Autodesk Inventor part; units mm, degrees
(part 2 of 2)
  point P149 (-1.693, 40.4752)
  point P150 (-1.6779, 40.4117)
  point P151 (-1.6594, 40.3487)
  point P152 (-5.9644, 41.4834)
  point P153 (-3.9838, 41.7202)
  point P154 (-4.0844, 40.3041)
  point P155 (-4.0904, 40.2391)
  point P156 (-4.0997, 40.1742)
  point P157 (-4.7872, 40.0384)
  point P158 (-5.5328, 40.131)
  point P159 (-5.5116, 40.0692)
  point P160 (-5.4872, 40.0083)
  point P161 (-9.8807, 40.7286)
  point P162 (-7.9315, 41.1526)
  point P163 (-7.8971, 39.7334)
  point P164 (-7.8968, 39.6681)
  point P165 (-7.9, 39.6025)
  point P166 (-9.3224, 39.4233)
  point P167 (-9.2955, 39.3638)
  point P168 (-9.2654, 39.3055)
  point P169 (-13.7074, 39.605)
  point P170 (-11.8074, 40.2124)
  point P171 (-11.6382, 38.8028)
  point P172 (-11.6318, 38.7378)
  point P173 (-11.6287, 38.6723)
  point P174 (-12.278, 38.4088)
  point P175 (-13.0276, 38.3587)
  point P176 (-12.9952, 38.302)
  point P177 (-12.9597, 38.2468)
  point P178 (-17.41, 38.1227)
  point P179 (-15.5764, 38.9079)
  point P180 (-15.274, 37.5208)
  point P181 (-15.2614, 37.4567)
  point P182 (-15.252, 37.3918)
  point P183 (-15.8734, 37.0678)
  point P184 (-16.6148, 36.9466)
  point P185 (-16.5772, 36.8933)
  point P186 (-16.5366, 36.8417)
  point P187 (-20.955, 36.2951)
  point P188 (-19.2043, 37.2511)
  point P189 (-18.7714, 35.899)
  point P190 (-18.7528, 35.8364)
  point P191 (-18.7373, 35.7727)
  point P192 (-19.325, 35.3911)
  point P193 (-20.0516, 35.2)
  point P194 (-20.009, 35.1505)
  point P195 (-19.9637, 35.103)
  point P196 (-24.3102, 34.1389)
  point P197 (-22.6583, 35.2569)
  point P198 (-22.0988, 33.9521)
  point P199 (-22.0743, 33.8916)
  dimension "d1" = 14.5
  dimension "d2" = 10.4934
  dimension "d12" = 75.5
  dimension "d15" = 40.3225
  dimension "d16" = 75.5
  dimension "d17" = 40.3225
  dimension "d18" = 75.5
  dimension "d19" = 40.3225
  dimension "d20" = 75.5
  dimension "d21" = 40.3225
  dimension "d23" = 10.4934
  dimension "d24" = 4.2774
  dimension "d26" = 1.364
  dimension "d27" = 14.7708
  dimension "d30" = 360
  constraints: 338 point on circle, 136 centre point, 36 end point, 7 symmetric about line, 6 point on line, 2 coincident, 2 equal length, 1 collinear, 1 horizontal, 1 horizontal alignment, 1 perpendicular, 1 tangent, 1 vertical, 2598 other
  measures "d1" angle of L0 L1
  measures "d2" distance of L1.end L0.end
  measures "d12" angle of L3 L5
  measures "d15" distance from line of point (0, 0) L3
  measures "d17" distance from line of point (0, 0) L6
  measures "d18" angle of L9 L10
  measures "d19" distance from line of point (0, 0) L9
  measures "d20" angle of L12 L13
  measures "d21" distance from line of L0.start L12
  measures "d26" angle of L0 L17
  measures "d27" distance of L16.start L16.end
extrude "Extrusion1" add sketch "Sketch1" along normal blind 9.525 contours S1 S0 A4 A7 S2 S3 A3 S260 S263 A137 A136 S262 S261 S256 S259 A135 A134 S258 S257 S252 S255 A133 A132 S254 S253 S248 S251 A131 A130 S250 S249 S244 S247 A129 A128 S246 S245 S240 S243 A127 A126 S242 S241 S236 S239 A125 A124 S238 S237 S232 S235 A123 A122 S234 S233 S228 S231 A121 A120 S230 S229 S224 S227 A119 A118 S226 S225 S220 S223 A117 A116 S222 S221 S216 S219 A115 A114 S218 S217 S212 S215 A113 A112 S214 S213 S208 S211 A111 A110 S210 S209 S204 S207 A109 A108 S206 S205 S200 S203 A107 A106 S202 S201 S196 S199 A105 A104 S198 S197 S192 S195 A103 A102 S194 S193 S188 S191 A101 A100 S190 S189 S184 S187 A99 A98 S186 S185 S180 S183 A97 A96 S182 S181 S176 S179 A95 A94 S178 S177 S172 S175 A93 A92 S174 S173 S168 S171 A91 A90 S170 S169 S164 S167 A89 A88 S166 S165 S160 S163 A87 A86 S162 S161 S156 S159 A85 A84 S158 S157 S152 S155 A83 A82 S154 S153 S148 S151 A81 A80 S150 S149 S144 S147 A79 A78 S146 S145 S140 S143 A77 A76 S142 S141 S136 S139 A75 A74 S138 S137 S132 S135 A73 A72 S134 S133 S128 S131 A71 A70 S130 S129 S124 S127 A69 A68 S126 S125 S120 S123 A67 A66 S122 S121 S116 S119 A65 A64 S118 S117 S112 S115 A63 A62 S114 S113 S108 S111 A61 A60 S110 S109 S104 S107 A59 A58 S106 S105 S100 S103 A57 A56 S102 S101 S96 S99 A55 A54 S98 S97 S92 S95 A53 A52 S94 S93 S88 S91 A51 A50 S90 S89 S84 S87 A49 A48 S86 S85 S80 S83 A47 A46 S82 S81 S76 S79 A45 A44 S78 S77 S72 S75 A43 A42 S74 S73 S68 S71 A41 A40 S70 S69 S64 S67 A39 A38 S66 S65 S60 S63 A37 A36 S62 S61 S56 S59 A35 A34 S58 S57 S52 S55 A33 A32 S54 S53 S48 S51 A31 A30 S50 S49 S44 S47 A29 A28 S46 S45 S40 S43 A27 A26 S42 S41 S36 S39 A25 A24 S38 S37 S32 S35 A23 A22 S34 S33 S28 S31 A21 A20 S30 S29 S24 S27 A19 A18 S26 S25 S20 S23 A17 A16 S22 S21 S16 S19 A15 A14 S18 S17 S12 S15 A13 A12 S14 S13 S8 S11 A11 A10 S10 S9 S4 S7 A9 A8 S6 S5
sketch "Sketch2" plane through (0, 9.525, 0) normal (0, 1, 0) x (1, 0, 0)
  line L0 (-6.35, 3.6662) -> (0, 7.3323)
  line L1 (0, 7.3323) -> (6.35, 3.6662)
  line L2 (6.35, 3.6662) -> (6.35, -3.6662)
  line L3 (6.35, -3.6662) -> (0, -7.3323)
  line L4 (0, -7.3323) -> (-6.35, -3.6662)
  line L5 (-6.35, -3.6662) -> (-6.35, 3.6662)
  point P0 (0, 0)
  point P1 (0, 0)
  dimension "d34" = 12.7
  constraints: 12 end point, 1 coincident, 1 vertical alignment, 13 other
  measures "d34" distance between parallel lines of L2 L5
sketch "Sketch4" plane through (0, 0, 0) normal (0, -1, 0) x (1, 0, 0)
  arc A0 (-40.3225, -0.2901) -> (-40.2906, -1.6288) centre (0, 0) ccw projected
  arc A1 (-43.11, -2.4585) -> (-43.021, -3.7017) centre (0, 0) ccw projected
  arc A2 (-40.1123, -4.1217) -> (-39.9534, -5.4513) centre (0, 0) ccw projected
  arc A3 (-42.6811, -6.5452) -> (-42.4744, -7.7743) centre (0, 0) ccw projected
  arc A4 (-39.5389, -7.916) -> (-39.2543, -9.2244) centre (0, 0) ccw projected
  arc A5 (-41.8656, -10.5727) -> (-41.543, -11.7766) centre (0, 0) ccw projected
  arc A6 (-38.6074, -11.6385) -> (-38.1997, -12.914) centre (0, 0) ccw projected
  arc A7 (-40.6711, -14.5044) -> (-40.2355, -15.6722) centre (0, 0) ccw projected
  arc A8 (-37.3263, -15.2557) -> (-36.7992, -16.4867) centre (0, 0) ccw projected
  arc A9 (-39.1082, -18.3048) -> (-38.5636, -19.4258) centre (0, 0) ccw projected
  arc A10 (-35.7071, -18.7347) -> (-35.0654, -19.91) centre (0, 0) ccw projected
  arc A11 (-37.1911, -21.9393) -> (-36.5424, -23.0036) centre (0, 0) ccw projected
  arc A12 (-33.7646, -22.0441) -> (-33.014, -23.153) centre (0, 0) ccw projected
  arc A13 (-34.9372, -25.3752) -> (-34.1903, -26.373) centre (0, 0) ccw projected
  arc A14 (-31.5163, -25.1538) -> (-30.6637, -26.1864) centre (0, 0) ccw projected
  arc A15 (-32.367, -28.5813) -> (-31.5286, -29.5036) centre (0, 0) ccw projected
  arc A16 (-28.9825, -28.0357) -> (-28.0357, -28.9825) centre (0, 0) ccw projected
  arc A17 (-29.5036, -31.5286) -> (-28.5813, -32.367) centre (0, 0) ccw projected
  arc A18 (-26.1864, -30.6637) -> (-25.1538, -31.5163) centre (0, 0) ccw projected
  arc A19 (-26.373, -34.1903) -> (-25.3752, -34.9372) centre (0, 0) ccw projected
  arc A20 (-23.153, -33.014) -> (-22.0441, -33.7646) centre (0, 0) ccw projected
  arc A21 (-23.0036, -36.5424) -> (-21.9393, -37.1911) centre (0, 0) ccw projected
  arc A22 (-19.91, -35.0654) -> (-18.7347, -35.7071) centre (0, 0) ccw projected
  arc A23 (-19.4258, -38.5636) -> (-18.3048, -39.1082) centre (0, 0) ccw projected
  arc A24 (-16.4867, -36.7992) -> (-15.2557, -37.3263) centre (0, 0) ccw projected
  arc A25 (-15.6722, -40.2355) -> (-14.5044, -40.6711) centre (0, 0) ccw projected
  arc A26 (-12.914, -38.1997) -> (-11.6385, -38.6074) centre (0, 0) ccw projected
  arc A27 (-11.7766, -41.543) -> (-10.5727, -41.8656) centre (0, 0) ccw projected
  arc A28 (-9.2244, -39.2543) -> (-7.916, -39.5389) centre (0, 0) ccw projected
  arc A29 (-7.7743, -42.4744) -> (-6.5452, -42.6811) centre (0, 0) ccw projected
  arc A30 (-5.4513, -39.9534) -> (-4.1217, -40.1123) centre (0, 0) ccw projected
  arc A31 (-3.7017, -43.021) -> (-2.4585, -43.11) centre (0, 0) ccw projected
  arc A32 (-1.6288, -40.2906) -> (-0.2901, -40.3225) centre (0, 0) ccw projected
  arc A33 (0.4045, -43.1781) -> (1.6505, -43.1484) centre (0, 0) ccw projected
  arc A34 (2.2084, -40.263) -> (3.5441, -40.1675) centre (0, 0) ccw projected
  arc A35 (4.507, -42.9441) -> (5.7445, -42.7962) centre (0, 0) ccw projected
  arc A36 (6.0257, -39.8708) -> (7.3462, -39.6487) centre (0, 0) ccw projected
  arc A37 (8.5687, -42.3213) -> (9.7866, -42.0563) centre (0, 0) ccw projected
  arc A38 (9.7883, -39.1175) -> (11.0818, -38.7709) centre (0, 0) ccw projected
  arc A39 (12.5528, -41.3151) -> (13.7399, -40.9356) centre (0, 0) ccw projected
  arc A40 (13.4624, -38.0099) -> (14.717, -37.5419) centre (0, 0) ccw projected
  arc A41 (16.4232, -39.9348) -> (17.5689, -39.4442) centre (0, 0) ccw projected
  arc A42 (17.0145, -36.5581) -> (18.219, -35.973) centre (0, 0) ccw projected
  arc A43 (20.1449, -38.1929) -> (21.2388, -37.5956) centre (0, 0) ccw projected
  arc A44 (20.4125, -34.7752) -> (21.5559, -34.0783) centre (0, 0) ccw projected
  arc A45 (23.6841, -36.1051) -> (24.7163, -35.4065) centre (0, 0) ccw projected
  arc A46 (23.6257, -32.6774) -> (24.6977, -31.875) centre (0, 0) ccw projected
  arc A47 (27.0089, -33.6903) -> (27.97, -32.8967) centre (0, 0) ccw projected
  arc A48 (26.6249, -30.2837) -> (27.6157, -29.383) centre (0, 0) ccw projected
  arc A49 (30.089, -30.9703) -> (30.9703, -30.089) centre (0, 0) ccw projected
  arc A50 (29.383, -27.6157) -> (30.2837, -26.6249) centre (0, 0) ccw projected
  arc A51 (32.8967, -27.97) -> (33.6903, -27.0089) centre (0, 0) ccw projected
  arc A52 (31.875, -24.6977) -> (32.6774, -23.6257) centre (0, 0) ccw projected
  arc A53 (35.4065, -24.7163) -> (36.1051, -23.6841) centre (0, 0) ccw projected
  arc A54 (34.0783, -21.5559) -> (34.7752, -20.4125) centre (0, 0) ccw projected
  arc A55 (37.5956, -21.2388) -> (38.1929, -20.1449) centre (0, 0) ccw projected
  arc A56 (35.973, -18.219) -> (36.5581, -17.0145) centre (0, 0) ccw projected
  arc A57 (39.4442, -17.5689) -> (39.9348, -16.4232) centre (0, 0) ccw projected
  arc A58 (37.5419, -14.717) -> (38.0099, -13.4624) centre (0, 0) ccw projected
  arc A59 (40.9356, -13.7399) -> (41.3151, -12.5528) centre (0, 0) ccw projected
  arc A60 (38.7709, -11.0818) -> (39.1175, -9.7883) centre (0, 0) ccw projected
  arc A61 (42.0563, -9.7866) -> (42.3213, -8.5687) centre (0, 0) ccw projected
  arc A62 (39.6487, -7.3462) -> (39.8708, -6.0257) centre (0, 0) ccw projected
  arc A63 (42.7962, -5.7445) -> (42.9441, -4.507) centre (0, 0) ccw projected
  arc A64 (40.1675, -3.5441) -> (40.263, -2.2084) centre (0, 0) ccw projected
  arc A65 (43.1484, -1.6505) -> (43.1781, -0.4045) centre (0, 0) ccw projected
  arc A66 (40.3225, 0.2901) -> (40.2906, 1.6288) centre (0, 0) ccw projected
  arc A67 (43.11, 2.4585) -> (43.021, 3.7017) centre (0, 0) ccw projected
  arc A68 (40.1123, 4.1217) -> (39.9534, 5.4513) centre (0, 0) ccw projected
  arc A69 (42.6811, 6.5452) -> (42.4744, 7.7743) centre (0, 0) ccw projected
  arc A70 (39.5389, 7.916) -> (39.2543, 9.2244) centre (0, 0) ccw projected
  arc A71 (41.8656, 10.5727) -> (41.543, 11.7766) centre (0, 0) ccw projected
  arc A72 (38.6074, 11.6385) -> (38.1997, 12.914) centre (0, 0) ccw projected
  arc A73 (40.6711, 14.5044) -> (40.2355, 15.6722) centre (0, 0) ccw projected
  arc A74 (37.3263, 15.2557) -> (36.7992, 16.4867) centre (0, 0) ccw projected
  arc A75 (39.1082, 18.3048) -> (38.5636, 19.4258) centre (0, 0) ccw projected
  arc A76 (35.7071, 18.7347) -> (35.0654, 19.91) centre (0, 0) ccw projected
  arc A77 (37.1911, 21.9393) -> (36.5424, 23.0036) centre (0, 0) ccw projected
  arc A78 (33.7646, 22.0441) -> (33.014, 23.153) centre (0, 0) ccw projected
  arc A79 (34.9372, 25.3752) -> (34.1903, 26.373) centre (0, 0) ccw projected
  arc A80 (31.5163, 25.1538) -> (30.6637, 26.1864) centre (0, 0) ccw projected
  arc A81 (32.367, 28.5813) -> (31.5286, 29.5036) centre (0, 0) ccw projected
  arc A82 (28.9825, 28.0357) -> (28.0357, 28.9825) centre (0, 0) ccw projected
  arc A83 (29.5036, 31.5286) -> (28.5813, 32.367) centre (0, 0) ccw projected
  arc A84 (26.1864, 30.6637) -> (25.1538, 31.5163) centre (0, 0) ccw projected
  arc A85 (26.373, 34.1903) -> (25.3752, 34.9372) centre (0, 0) ccw projected
  arc A86 (23.153, 33.014) -> (22.0441, 33.7646) centre (0, 0) ccw projected
  arc A87 (23.0036, 36.5424) -> (21.9393, 37.1911) centre (0, 0) ccw projected
  arc A88 (19.91, 35.0654) -> (18.7347, 35.7071) centre (0, 0) ccw projected
  arc A89 (19.4258, 38.5636) -> (18.3048, 39.1082) centre (0, 0) ccw projected
  arc A90 (16.4867, 36.7992) -> (15.2557, 37.3263) centre (0, 0) ccw projected
  arc A91 (15.6722, 40.2355) -> (14.5044, 40.6711) centre (0, 0) ccw projected
  arc A92 (12.914, 38.1997) -> (11.6385, 38.6074) centre (0, 0) ccw projected
  arc A93 (11.7766, 41.543) -> (10.5727, 41.8656) centre (0, 0) ccw projected
  arc A94 (9.2244, 39.2543) -> (7.916, 39.5389) centre (0, 0) ccw projected
  arc A95 (7.7743, 42.4744) -> (6.5452, 42.6811) centre (0, 0) ccw projected
  arc A96 (5.4513, 39.9534) -> (4.1217, 40.1123) centre (0, 0) ccw projected
  arc A97 (3.7017, 43.021) -> (2.4585, 43.11) centre (0, 0) ccw projected
  arc A98 (1.6288, 40.2906) -> (0.2901, 40.3225) centre (0, 0) ccw projected
  arc A99 (-0.4045, 43.1781) -> (-1.6505, 43.1484) centre (0, 0) ccw projected
  arc A100 (-2.2084, 40.263) -> (-3.5441, 40.1675) centre (0, 0) ccw projected
  arc A101 (-4.507, 42.9441) -> (-5.7445, 42.7962) centre (0, 0) ccw projected
  arc A102 (-6.0257, 39.8708) -> (-7.3462, 39.6487) centre (0, 0) ccw projected
  arc A103 (-8.5687, 42.3213) -> (-9.7866, 42.0563) centre (0, 0) ccw projected
  arc A104 (-9.7883, 39.1175) -> (-11.0818, 38.7709) centre (0, 0) ccw projected
  arc A105 (-12.5528, 41.3151) -> (-13.7399, 40.9356) centre (0, 0) ccw projected
  arc A106 (-13.4624, 38.0099) -> (-14.717, 37.5419) centre (0, 0) ccw projected
  arc A107 (-16.4232, 39.9348) -> (-17.5689, 39.4442) centre (0, 0) ccw projected
  arc A108 (-17.0145, 36.5581) -> (-18.219, 35.973) centre (0, 0) ccw projected
  arc A109 (-20.1449, 38.1929) -> (-21.2388, 37.5956) centre (0, 0) ccw projected
  arc A110 (-20.4125, 34.7752) -> (-21.5559, 34.0783) centre (0, 0) ccw projected
  arc A111 (-23.6841, 36.1051) -> (-24.7163, 35.4065) centre (0, 0) ccw projected
  arc A112 (-23.6257, 32.6774) -> (-24.6977, 31.875) centre (0, 0) ccw projected
  arc A113 (-27.0089, 33.6903) -> (-27.97, 32.8967) centre (0, 0) ccw projected
  arc A114 (-26.6249, 30.2837) -> (-27.6157, 29.383) centre (0, 0) ccw projected
  arc A115 (-30.089, 30.9703) -> (-30.9703, 30.089) centre (0, 0) ccw projected
  arc A116 (-29.383, 27.6157) -> (-30.2837, 26.6249) centre (0, 0) ccw projected
  arc A117 (-32.8967, 27.97) -> (-33.6903, 27.0089) centre (0, 0) ccw projected
  arc A118 (-31.875, 24.6977) -> (-32.6774, 23.6257) centre (0, 0) ccw projected
  arc A119 (-35.4065, 24.7163) -> (-36.1051, 23.6841) centre (0, 0) ccw projected
  arc A120 (-34.0783, 21.5559) -> (-34.7752, 20.4125) centre (0, 0) ccw projected
  arc A121 (-37.5956, 21.2388) -> (-38.1929, 20.1449) centre (0, 0) ccw projected
  arc A122 (-35.973, 18.219) -> (-36.5581, 17.0145) centre (0, 0) ccw projected
  arc A123 (-39.4442, 17.5689) -> (-39.9348, 16.4232) centre (0, 0) ccw projected
  arc A124 (-37.5419, 14.717) -> (-38.0099, 13.4624) centre (0, 0) ccw projected
  arc A125 (-40.9356, 13.7399) -> (-41.3151, 12.5528) centre (0, 0) ccw projected
  arc A126 (-38.7709, 11.0818) -> (-39.1175, 9.7883) centre (0, 0) ccw projected
  arc A127 (-42.0563, 9.7866) -> (-42.3213, 8.5687) centre (0, 0) ccw projected
  arc A128 (-39.6487, 7.3462) -> (-39.8708, 6.0257) centre (0, 0) ccw projected
  arc A129 (-42.7962, 5.7445) -> (-42.9441, 4.507) centre (0, 0) ccw projected
  arc A130 (-40.1675, 3.5441) -> (-40.263, 2.2084) centre (0, 0) ccw projected
  arc A131 (-43.1484, 1.6505) -> (-43.1781, 0.4045) centre (0, 0) ccw projected
  circle A132 centre (0, 0) radius 19.1008 construction
  line L0 (0, 0) -> (18.2308, 0) construction
  arc A133 (18.226, -0.4165) -> (18.2308, 0) centre (0, 0) ccw
  arc A134 (17.732, -0.8319) -> (18.226, -0.4165) centre (17.7962, -0.4067) ccw
  line L1 (0, 0) -> (17.5097, -2.3052) construction
  arc A135 (17.732, -0.8319) -> (16.0325, -2.1107) centre (17.5097, -2.3052) ccw
  line L2 (18.2308, 0) -> (19.1008, 0) construction
  line L3 (18.9374, -2.4932) -> (18.9042, -2.745) construction
  arc A136 (17.6096, -4.7185) -> (17.7128, -4.3149) centre (0, 0) ccw
  arc A137 (17.7128, -4.3149) -> (17.3431, -3.7859) centre (17.295, -4.2132) ccw
  arc A138 (16.0325, -2.1107) -> (17.3431, -3.7859) centre (17.5097, -2.3052) ccw
  line L4 (17.6096, -4.7185) -> (18.45, -4.9437) construction
  arc A139 (17.7128, 4.3149) -> (17.6096, 4.7185) centre (0, 0) ccw
  arc A140 (17.3431, 3.7859) -> (17.7128, 4.3149) centre (17.295, 4.2132) ccw
  arc A141 (17.3431, 3.7859) -> (16.0325, 2.1107) centre (17.5097, 2.3052) ccw
  arc A142 (16.0325, 2.1107) -> (17.732, 0.8319) centre (17.5097, 2.3052) ccw
  arc A143 (18.226, 0.4165) -> (17.732, 0.8319) centre (17.7962, 0.4067) ccw
  arc A144 (18.2308, 0) -> (18.226, 0.4165) centre (0, 0) ccw
  arc A145 (15.9925, 8.7523) -> (15.7883, 9.1154) centre (0, 0) ccw
  arc A146 (15.7723, 8.1456) -> (15.9925, 8.7523) centre (15.6153, 8.5459) ccw
  arc A147 (15.7723, 8.1456) -> (14.9399, 6.1883) centre (16.3165, 6.7585) ccw
  arc A148 (14.9399, 6.1883) -> (16.9125, 5.3929) centre (16.3165, 6.7585) ccw
  arc A149 (17.4972, 5.1196) -> (16.9125, 5.3929) centre (17.0845, 4.9988) ccw
  arc A150 (17.6096, 4.7185) -> (17.4972, 5.1196) centre (0, 0) ccw
  arc A151 (13.1823, 12.5932) -> (12.8911, 12.8911) centre (0, 0) ccw
  arc A152 (13.1266, 11.9502) -> (13.1823, 12.5932) centre (12.8714, 12.2962) ccw
  arc A153 (13.1266, 11.9502) -> (12.8292, 9.8442) centre (14.0113, 10.7512) ccw
  arc A154 (12.8292, 9.8442) -> (14.9404, 9.5864) centre (14.0113, 10.7512) ccw
  arc A155 (15.576, 9.4737) -> (14.9404, 9.5864) centre (15.2086, 9.2503) ccw
  arc A156 (15.7883, 9.1154) -> (15.576, 9.4737) centre (0, 0) ccw
  arc A157 (9.4737, 15.576) -> (9.1154, 15.7883) centre (0, 0) ccw
  arc A158 (9.5864, 14.9404) -> (9.4737, 15.576) centre (9.2503, 15.2086) ccw
  arc A159 (9.5864, 14.9404) -> (9.8442, 12.8292) centre (10.7512, 14.0113) ccw
  arc A160 (9.8442, 12.8292) -> (11.9502, 13.1266) centre (10.7512, 14.0113) ccw
  arc A161 (12.5932, 13.1823) -> (11.9502, 13.1266) centre (12.2962, 12.8714) ccw
  arc A162 (12.8911, 12.8911) -> (12.5932, 13.1823) centre (0, 0) ccw
  arc A163 (5.1196, 17.4972) -> (4.7185, 17.6096) centre (0, 0) ccw
  arc A164 (5.3929, 16.9125) -> (5.1196, 17.4972) centre (4.9988, 17.0845) ccw
  arc A165 (5.3929, 16.9125) -> (6.1883, 14.9399) centre (6.7585, 16.3165) ccw
  arc A166 (6.1883, 14.9399) -> (8.1456, 15.7723) centre (6.7585, 16.3165) ccw
  arc A167 (8.7523, 15.9925) -> (8.1456, 15.7723) centre (8.5459, 15.6153) ccw
  arc A168 (9.1154, 15.7883) -> (8.7523, 15.9925) centre (0, 0) ccw
  arc A169 (0.4165, 18.226) -> (0, 18.2308) centre (0, 0) ccw
  arc A170 (0.8319, 17.732) -> (0.4165, 18.226) centre (0.4067, 17.7962) ccw
  arc A171 (0.8319, 17.732) -> (2.1107, 16.0325) centre (2.3052, 17.5097) ccw
  arc A172 (2.1107, 16.0325) -> (3.7859, 17.3431) centre (2.3052, 17.5097) ccw
  arc A173 (4.3149, 17.7128) -> (3.7859, 17.3431) centre (4.2132, 17.295) ccw
  arc A174 (4.7185, 17.6096) -> (4.3149, 17.7128) centre (0, 0) ccw
  arc A175 (-4.3149, 17.7128) -> (-4.7185, 17.6096) centre (0, 0) ccw
  arc A176 (-3.7859, 17.3431) -> (-4.3149, 17.7128) centre (-4.2132, 17.295) ccw
  arc A177 (-3.7859, 17.3431) -> (-2.1107, 16.0325) centre (-2.3052, 17.5097) ccw
  arc A178 (-2.1107, 16.0325) -> (-0.8319, 17.732) centre (-2.3052, 17.5097) ccw
  arc A179 (-0.4165, 18.226) -> (-0.8319, 17.732) centre (-0.4067, 17.7962) ccw
  arc A180 (0, 18.2308) -> (-0.4165, 18.226) centre (0, 0) ccw
  arc A181 (-8.7523, 15.9925) -> (-9.1154, 15.7883) centre (0, 0) ccw
  arc A182 (-8.1456, 15.7723) -> (-8.7523, 15.9925) centre (-8.5459, 15.6153) ccw
  arc A183 (-8.1456, 15.7723) -> (-6.1883, 14.9399) centre (-6.7585, 16.3165) ccw
  arc A184 (-6.1883, 14.9399) -> (-5.3929, 16.9125) centre (-6.7585, 16.3165) ccw
  arc A185 (-5.1196, 17.4972) -> (-5.3929, 16.9125) centre (-4.9988, 17.0845) ccw
  arc A186 (-4.7185, 17.6096) -> (-5.1196, 17.4972) centre (0, 0) ccw
  arc A187 (-12.5932, 13.1823) -> (-12.8911, 12.8911) centre (0, 0) ccw
  arc A188 (-11.9502, 13.1266) -> (-12.5932, 13.1823) centre (-12.2962, 12.8714) ccw
  arc A189 (-11.9502, 13.1266) -> (-9.8442, 12.8292) centre (-10.7512, 14.0113) ccw
  arc A190 (-9.8442, 12.8292) -> (-9.5864, 14.9404) centre (-10.7512, 14.0113) ccw
  arc A191 (-9.4737, 15.576) -> (-9.5864, 14.9404) centre (-9.2503, 15.2086) ccw
  arc A192 (-9.1154, 15.7883) -> (-9.4737, 15.576) centre (0, 0) ccw
  arc A193 (-15.576, 9.4737) -> (-15.7883, 9.1154) centre (0, 0) ccw
  arc A194 (-14.9404, 9.5864) -> (-15.576, 9.4737) centre (-15.2086, 9.2503) ccw
  arc A195 (-14.9404, 9.5864) -> (-12.8292, 9.8442) centre (-14.0113, 10.7512) ccw
  arc A196 (-12.8292, 9.8442) -> (-13.1266, 11.9502) centre (-14.0113, 10.7512) ccw
  arc A197 (-13.1823, 12.5932) -> (-13.1266, 11.9502) centre (-12.8714, 12.2962) ccw
  arc A198 (-12.8911, 12.8911) -> (-13.1823, 12.5932) centre (0, 0) ccw
  arc A199 (-17.4972, 5.1196) -> (-17.6096, 4.7185) centre (0, 0) ccw
  arc A200 (-16.9125, 5.3929) -> (-17.4972, 5.1196) centre (-17.0845, 4.9988) ccw
  arc A201 (-16.9125, 5.3929) -> (-14.9399, 6.1883) centre (-16.3165, 6.7585) ccw
  arc A202 (-14.9399, 6.1883) -> (-15.7723, 8.1456) centre (-16.3165, 6.7585) ccw
  arc A203 (-15.9925, 8.7523) -> (-15.7723, 8.1456) centre (-15.6153, 8.5459) ccw
  arc A204 (-15.7883, 9.1154) -> (-15.9925, 8.7523) centre (0, 0) ccw
  arc A205 (-18.226, 0.4165) -> (-18.2308, 0) centre (0, 0) ccw
  arc A206 (-17.732, 0.8319) -> (-18.226, 0.4165) centre (-17.7962, 0.4067) ccw
  arc A207 (-17.732, 0.8319) -> (-16.0325, 2.1107) centre (-17.5097, 2.3052) ccw
  arc A208 (-16.0325, 2.1107) -> (-17.3431, 3.7859) centre (-17.5097, 2.3052) ccw
  arc A209 (-17.7128, 4.3149) -> (-17.3431, 3.7859) centre (-17.295, 4.2132) ccw
  arc A210 (-17.6096, 4.7185) -> (-17.7128, 4.3149) centre (0, 0) ccw
  arc A211 (-17.7128, -4.3149) -> (-17.6096, -4.7185) centre (0, 0) ccw
  arc A212 (-17.3431, -3.7859) -> (-17.7128, -4.3149) centre (-17.295, -4.2132) ccw
  arc A213 (-17.3431, -3.7859) -> (-16.0325, -2.1107) centre (-17.5097, -2.3052) ccw
  arc A214 (-16.0325, -2.1107) -> (-17.732, -0.8319) centre (-17.5097, -2.3052) ccw
  arc A215 (-18.226, -0.4165) -> (-17.732, -0.8319) centre (-17.7962, -0.4067) ccw
  arc A216 (-18.2308, 0) -> (-18.226, -0.4165) centre (0, 0) ccw
  arc A217 (-15.9925, -8.7523) -> (-15.7883, -9.1154) centre (0, 0) ccw
  arc A218 (-15.7723, -8.1456) -> (-15.9925, -8.7523) centre (-15.6153, -8.5459) ccw
  arc A219 (-15.7723, -8.1456) -> (-14.9399, -6.1883) centre (-16.3165, -6.7585) ccw
  arc A220 (-14.9399, -6.1883) -> (-16.9125, -5.3929) centre (-16.3165, -6.7585) ccw
  arc A221 (-17.4972, -5.1196) -> (-16.9125, -5.3929) centre (-17.0845, -4.9988) ccw
  arc A222 (-17.6096, -4.7185) -> (-17.4972, -5.1196) centre (0, 0) ccw
  arc A223 (-13.1823, -12.5932) -> (-12.8911, -12.8911) centre (0, 0) ccw
  arc A224 (-13.1266, -11.9502) -> (-13.1823, -12.5932) centre (-12.8714, -12.2962) ccw
  arc A225 (-13.1266, -11.9502) -> (-12.8292, -9.8442) centre (-14.0113, -10.7512) ccw
  arc A226 (-12.8292, -9.8442) -> (-14.9404, -9.5864) centre (-14.0113, -10.7512) ccw
  arc A227 (-15.576, -9.4737) -> (-14.9404, -9.5864) centre (-15.2086, -9.2503) ccw
  arc A228 (-15.7883, -9.1154) -> (-15.576, -9.4737) centre (0, 0) ccw
  arc A229 (-9.4737, -15.576) -> (-9.1154, -15.7883) centre (0, 0) ccw
  arc A230 (-9.5864, -14.9404) -> (-9.4737, -15.576) centre (-9.2503, -15.2086) ccw
  arc A231 (-9.5864, -14.9404) -> (-9.8442, -12.8292) centre (-10.7512, -14.0113) ccw
  arc A232 (-9.8442, -12.8292) -> (-11.9502, -13.1266) centre (-10.7512, -14.0113) ccw
  arc A233 (-12.5932, -13.1823) -> (-11.9502, -13.1266) centre (-12.2962, -12.8714) ccw
  arc A234 (-12.8911, -12.8911) -> (-12.5932, -13.1823) centre (0, 0) ccw
  arc A235 (-5.1196, -17.4972) -> (-4.7185, -17.6096) centre (0, 0) ccw
  arc A236 (-5.3929, -16.9125) -> (-5.1196, -17.4972) centre (-4.9988, -17.0845) ccw
  arc A237 (-5.3929, -16.9125) -> (-6.1883, -14.9399) centre (-6.7585, -16.3165) ccw
  arc A238 (-6.1883, -14.9399) -> (-8.1456, -15.7723) centre (-6.7585, -16.3165) ccw
  arc A239 (-8.7523, -15.9925) -> (-8.1456, -15.7723) centre (-8.5459, -15.6153) ccw
  arc A240 (-9.1154, -15.7883) -> (-8.7523, -15.9925) centre (0, 0) ccw
  arc A241 (-0.4165, -18.226) -> (0, -18.2308) centre (0, 0) ccw
  arc A242 (-0.8319, -17.732) -> (-0.4165, -18.226) centre (-0.4067, -17.7962) ccw
  arc A243 (-0.8319, -17.732) -> (-2.1107, -16.0325) centre (-2.3052, -17.5097) ccw
  arc A244 (-2.1107, -16.0325) -> (-3.7859, -17.3431) centre (-2.3052, -17.5097) ccw
  arc A245 (-4.3149, -17.7128) -> (-3.7859, -17.3431) centre (-4.2132, -17.295) ccw
  arc A246 (-4.7185, -17.6096) -> (-4.3149, -17.7128) centre (0, 0) ccw
  arc A247 (4.3149, -17.7128) -> (4.7185, -17.6096) centre (0, 0) ccw
  arc A248 (3.7859, -17.3431) -> (4.3149, -17.7128) centre (4.2132, -17.295) ccw
  arc A249 (3.7859, -17.3431) -> (2.1107, -16.0325) centre (2.3052, -17.5097) ccw
  arc A250 (2.1107, -16.0325) -> (0.8319, -17.732) centre (2.3052, -17.5097) ccw
  arc A251 (0.4165, -18.226) -> (0.8319, -17.732) centre (0.4067, -17.7962) ccw
  arc A252 (0, -18.2308) -> (0.4165, -18.226) centre (0, 0) ccw
  arc A253 (8.7523, -15.9925) -> (9.1154, -15.7883) centre (0, 0) ccw
  arc A254 (8.1456, -15.7723) -> (8.7523, -15.9925) centre (8.5459, -15.6153) ccw
  arc A255 (8.1456, -15.7723) -> (6.1883, -14.9399) centre (6.7585, -16.3165) ccw
  arc A256 (6.1883, -14.9399) -> (5.3929, -16.9125) centre (6.7585, -16.3165) ccw
  arc A257 (5.1196, -17.4972) -> (5.3929, -16.9125) centre (4.9988, -17.0845) ccw
  arc A258 (4.7185, -17.6096) -> (5.1196, -17.4972) centre (0, 0) ccw
  arc A259 (12.5932, -13.1823) -> (12.8911, -12.8911) centre (0, 0) ccw
  arc A260 (11.9502, -13.1266) -> (12.5932, -13.1823) centre (12.2962, -12.8714) ccw
  arc A261 (11.9502, -13.1266) -> (9.8442, -12.8292) centre (10.7512, -14.0113) ccw
  arc A262 (9.8442, -12.8292) -> (9.5864, -14.9404) centre (10.7512, -14.0113) ccw
  arc A263 (9.4737, -15.576) -> (9.5864, -14.9404) centre (9.2503, -15.2086) ccw
  arc A264 (9.1154, -15.7883) -> (9.4737, -15.576) centre (0, 0) ccw
  arc A265 (15.576, -9.4737) -> (15.7883, -9.1154) centre (0, 0) ccw
  arc A266 (14.9404, -9.5864) -> (15.576, -9.4737) centre (15.2086, -9.2503) ccw
  arc A267 (14.9404, -9.5864) -> (12.8292, -9.8442) centre (14.0113, -10.7512) ccw
  arc A268 (12.8292, -9.8442) -> (13.1266, -11.9502) centre (14.0113, -10.7512) ccw
  arc A269 (13.1823, -12.5932) -> (13.1266, -11.9502) centre (12.8714, -12.2962) ccw
  arc A270 (12.8911, -12.8911) -> (13.1823, -12.5932) centre (0, 0) ccw
  arc A271 (17.4972, -5.1196) -> (17.6096, -4.7185) centre (0, 0) ccw
  arc A272 (16.9125, -5.3929) -> (17.4972, -5.1196) centre (17.0845, -4.9988) ccw
  arc A273 (16.9125, -5.3929) -> (14.9399, -6.1883) centre (16.3165, -6.7585) ccw
  arc A274 (14.9399, -6.1883) -> (15.7723, -8.1456) centre (16.3165, -6.7585) ccw
  arc A275 (15.9925, -8.7523) -> (15.7723, -8.1456) centre (15.6153, -8.5459) ccw
  arc A276 (15.7883, -9.1154) -> (15.9925, -8.7523) centre (0, 0) ccw
  point P0 (18.2308, 0)
  point P1 (17.6096, 4.7185)
  point P2 (15.7883, 9.1154)
  point P3 (9.1154, 15.7883)
  point P4 (4.7185, 17.6096)
  point P5 (0, 18.2308)
  point P6 (-4.7185, 17.6096)
  point P7 (-9.1154, 15.7883)
  point P8 (-12.8911, 12.8911)
  point P9 (-15.7883, 9.1154)
  point P10 (-17.6096, 4.7185)
  point P11 (-18.2308, 0)
  point P12 (-17.6096, -4.7185)
  point P13 (-15.7883, -9.1154)
  point P14 (-12.8911, -12.8911)
  point P15 (-9.1154, -15.7883)
  point P16 (-4.7185, -17.6096)
  point P17 (0, -18.2308)
  point P18 (4.7185, -17.6096)
  point P19 (9.1154, -15.7883)
  point P20 (12.8911, -12.8911)
  point P21 (15.7883, -9.1154)
  dimension "d41" = 38.2016
  dimension "d43" = 0.43
  dimension "d44" = 1.49
  dimension "d45" = 0.87
  dimension "d46" = 2.93
  dimension "d47" = 0.254
  dimension "d48" = 7.5
  dimension "d55" = 360
  constraints: 290 point on circle, 145 centre point, 10 end point, 5 symmetric about line, 3 tangent, 2 coincident, 2 horizontal, 2 point on line, 1 concentric, 676 other
  measures "d41" diameter of A132
  measures "d43" radius of A134
  measures "d44" radius of A135
  measures "d45" distance of L0.end L2.end
  measures "d46" distance from line of A135.end L3
  measures "d47" distance of L3.start L3.end
  measures "d48" angle of L0 L1
extrude "Extrusion4" add sketch "Sketch4" along normal blind 10
sketch "Sketch5" plane through (0, -10, 0) normal (0, -1, 0) x (1, 0, 0)
  circle A0 centre (0, 0) radius 19.1008
  dimension "d59" = 38.2016
  constraints: 1 centre point, 1 coincident
  measures "d59" diameter of A0
extrude "Extrusion5" add sketch "Sketch5" along normal blind 0.635
extrude "Extrusion7" cut sketch "Sketch2" along normal through all both and the other way through all
sketch "Sketch6" plane through (0, 9.525, 0) normal (0, 1, 0) x (1, 0, 0)
  circle A0 centre (0, 0) radius 8.89
  line L0 (-6.35, 3.6662) -> (0, 7.3323)
  line L1 (0, 7.3323) -> (6.35, 3.6662)
  line L2 (6.35, 3.6662) -> (6.35, -3.6662)
  line L3 (6.35, -3.6662) -> (0, -7.3323)
  line L4 (0, -7.3323) -> (-6.35, -3.6662)
  line L5 (-6.35, -3.6662) -> (-6.35, 3.6662)
  dimension "d66" = 17.78
  dimension "d67" = 12.7
  dimension "d68" = 3.6662
  constraints: 12 end point, 2 coincident, 1 centre point, 13 other
  measures "d66" diameter of A0
  measures "d67" distance between parallel lines of L2 L5
  measures "d68" vertical distance of A0.centre L4.end
extrude "Extrusion8" add sketch "Sketch6" along normal blind 2.794
body "Solid1"
